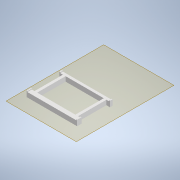
# Autodesk Inventor part: display_holder
Saved by Autodesk Inventor 2022 (Build 260153000, 153)
## iProperties
Created: 2021-12-06
Part Number: display_holder
Material: Generic
Document SubType Name: Modeling
Designer: simen
Density: 1 g/cm^3
Appearance: Default
Author: simen
## iProperties of the stored document display_holder_3DPrint.ipt
Created: 2021-12-08
Part Number: display_holder_3DPrint
Material: Generic
Document SubType Name: Modeling
Designer: simen
Density: 1 g/cm^3
Appearance: Default
Author: simen
Autodesk Inventor part; units mm, degrees
ref_plane "YZ Plane" through (0, 0, 0) normal (1, 0, 0) x (0, 1, 0)
ref_plane "XZ Plane" through (0, 0, 0) normal (0, 1, 0) x (-1, 0, 0)
ref_plane "XY Plane" through (0, 0, 0) normal (0, 0, 1) x (1, 0, 0)
ref_plane "Work Plane1" through (-15.1761, -6.8152, -116.1136) normal (0, 1, 0) x (0, 0, -1)
sketch "Sketch6" plane through (-15.1761, -6.8152, -116.1136) normal (0, 1, 0) x (0, 0, -1)
  line L0 (-86.4323, 1.0655) -> (-81.4323, 1.0655)
  line L1 (-81.4323, -55.9345) -> (-86.4323, -55.9345)
  line L2 (-86.4323, -55.9345) -> (-86.4323, 1.0655)
  line L3 (-49.4323, 1.0655) -> (-46.4323, 1.0655)
  line L4 (-46.4323, 1.0655) -> (-46.4323, -55.9345)
  line L5 (-46.4323, -55.9345) -> (-49.4323, -55.9345)
  line L6 (-81.4323, -48.9345) -> (-49.4323, -48.9345)
  line L7 (-49.4323, -51.9345) -> (-81.4323, -51.9345)
  line L8 (-81.4323, -2.9345) -> (-49.4323, -2.9345)
  line L9 (-49.4323, -5.9345) -> (-81.4323, -5.9345)
  line L10 (-81.4323, 1.0655) -> (-81.4323, -2.9345)
  line L11 (-49.4323, -2.9345) -> (-49.4323, 1.0655)
  line L12 (-49.4323, -55.9345) -> (-49.4323, -51.9345)
  line L13 (-49.4323, -48.9345) -> (-49.4323, -5.9345)
  line L14 (-81.4323, -5.9345) -> (-81.4323, -48.9345)
  line L15 (-81.4323, -51.9345) -> (-81.4323, -55.9345)
  point P0 (-116.1136, -15.1761)
  dimension "d15" = 5
  dimension "d16" = 57
  dimension "d18" = 3
  dimension "d19" = 57
  dimension "d20" = 3
  dimension "d21" = 3
  dimension "d24" = 4
  dimension "d25" = 4
  dimension "d26" = 32
  dimension "d27" = 40
  constraints: 32 end point, 10 parallel, 4 horizontal, 4 perpendicular, 1 collinear
  measures "d15" distance of L1.start L1.end
  measures "d16" distance of L0.end L1.start
  measures "d18" distance of L4.end L5.end
  measures "d19" distance of L4.start L4.end
  measures "d20" distance between parallel lines of L6 L7
  measures "d21" distance between parallel lines of L8 L9
  measures "d24" distance of L7.end L1.start
  measures "d25" distance of L0.end L8.start
  measures "d26" distance between parallel lines of L13 L14
  measures "d27" distance between parallel lines of L4 L2
extrude "Extrusion6" add sketch "Sketch6" along normal blind 5.2
sketch "Sketch7" plane through (-15.1761, -1.6152, -116.1136) normal (0, 1, 0) x (1, 0, 0)
  line L0 (55.9345, -86.4323) -> (55.9345, -81.4323) projected
  line L1 (55.9345, -81.4323) -> (51.9345, -81.4323) projected
  line L2 (51.9345, -81.4323) -> (51.9345, -49.4323) projected
  line L3 (51.9345, -49.4323) -> (55.9345, -49.4323) projected
  line L4 (55.9345, -49.4323) -> (55.9345, -46.4323) projected
  line L5 (55.9345, -46.4323) -> (-1.0655, -46.4323) projected
  line L6 (-1.0655, -46.4323) -> (-1.0655, -49.4323) projected
  line L7 (-1.0655, -49.4323) -> (2.9345, -49.4323) projected
  line L8 (2.9345, -49.4323) -> (2.9345, -81.4323) projected
  line L9 (2.9345, -81.4323) -> (-1.0655, -81.4323) projected
  line L10 (-1.0655, -81.4323) -> (-1.0655, -86.4323) projected
  line L11 (-1.0655, -86.4323) -> (55.9345, -86.4323) projected
  line L12 (48.9345, -81.4323) -> (5.9345, -81.4323) projected
  line L13 (5.9345, -81.4323) -> (5.9345, -49.4323) projected
  line L14 (5.9345, -49.4323) -> (48.9345, -49.4323) projected
  line L15 (48.9345, -49.4323) -> (48.9345, -81.4323) projected
  line L16 (-1.0655, -86.4323) -> (55.9345, -86.4323) projected
  line L17 (-0.0655, -86.4323) -> (-0.0655, -81.4323)
  line L18 (-0.0655, -49.4323) -> (-0.0655, -46.4323)
  line L19 (54.9345, -86.4323) -> (54.9345, -81.4323)
  line L20 (55.9345, -81.4323) -> (51.9345, -81.4323) projected
  line L21 (51.9345, -49.4323) -> (55.9345, -49.4323) projected
  line L22 (54.9345, -49.4323) -> (54.9345, -46.4323)
  point P0 (15.1761, -116.1136)
  point P1 (54.9345, -49.4323)
  point P2 (-0.0655, -86.4323)
  dimension "d30" = 1
  dimension "d31" = 1
  dimension "d32" = 1
  dimension "d33" = 1
  constraints: 8 end point, 8 point on line, 3 perpendicular, 1 parallel
  measures "d30" distance between parallel lines of L4 L22
  measures "d31" distance between parallel lines of L0 L19
  measures "d32" distance between parallel lines of L10 L17
  measures "d33" distance between parallel lines of L6 L18
extrude "Extrusion7" add sketch "Sketch7" along normal blind 1 contours L11 L19 L1 L0 | L11 L10 L9 L17 | L22 L5 L4 L3 | L7 L6 L5 L18
body "Solid2"
